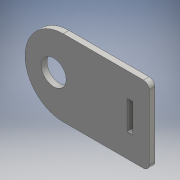
# Autodesk Inventor part: sample_mount
Saved by Autodesk Inventor 2016 (Build 200138000, 138)
## iProperties
Created: 2018-10-08
Part Number: sample_mount
Material: Generic
Document SubType Name: Modeling
Designer: andrew
Density: 1 g/cm^3
Appearance: Default
Author: andrew
Autodesk Inventor part; units mm, degrees
ref_plane "YZ Plane" through (0, 0, 0) normal (1, 0, 0) x (0, 1, 0)
ref_plane "XZ Plane" through (0, 0, 0) normal (0, 1, 0) x (-1, 0, 0)
ref_plane "XY Plane" through (0, 0, 0) normal (0, 0, 1) x (1, 0, 0)
sketch "Sketch1" plane through (0, 0, 0) normal (0, 1, 0) x (-1, 0, 0)
  line L0 (-22.5, 20) -> (22.5, 20)
  line L1 (22.5, 20) -> (22.5, -20)
  line L2 (22.5, -20) -> (-22.5, -20)
  line L3 (-22.5, -20) -> (-22.5, 20)
  line L4 (-22.5, 20) -> (22.5, -20) construction
  line L5 (22.5, 20) -> (-22.5, -20) construction
  arc A0 (22.5, -20) -> (22.5, 20) centre (22.5, 0) ccw
  point P0 (0, 0)
  dimension "d0" = 45
  dimension "d1" = 40
  dimension "d2" = 20
  constraints: 12 end point, 2 midpoint, 2 parallel, 2 point on circle, 1 centre point, 1 horizontal, 1 perpendicular
  measures "d0" distance of L1.end L2.end
  measures "d1" distance of L0.end L1.end
  measures "d2" radius of A0
extrude "Extrusion1" add sketch "Sketch1" along normal blind 3
sketch "Sketch2" plane through (0, 3, 0) normal (0, 1, 0) x (1, 0, 0)
  arc A0 (-22.5, 20) -> (-22.5, -20) centre (-22.5, 0) ccw construction
  line L0 (-42.5, 0) -> (-27.5, 0) construction
  point P0 (0, 0)
  dimension "d5" = 15
  constraints: 2 end point, 1 coincident, 1 horizontal, 1 point on circle
  measures "d5" distance of L0.start L0.end
hole "Hole1" at (-27.5, 3, 0) direction (0, -1, 0) diameter 13 end through all
sketch "Sketch4" plane through (0, 0, 0) normal (0, -1, 0) x (1, 0, 0)
  line L0 (22.5, 20) -> (22.5, -20) construction
  line L1 (22.5, 0) -> (12.5, 0) construction
  line L2 (11, -7.5) -> (14, -7.5)
  line L3 (14, -7.5) -> (14, 7.5)
  line L4 (14, 7.5) -> (11, 7.5)
  line L5 (11, 7.5) -> (11, -7.5)
  line L6 (11, -7.5) -> (14, 7.5) construction
  line L7 (14, -7.5) -> (11, 7.5) construction
  point P0 (0, 0)
  dimension "d17" = 10
  dimension "d18" = 3
  dimension "d19" = 15
  constraints: 14 end point, 3 midpoint, 2 horizontal, 2 parallel, 1 perpendicular
  measures "d17" distance of L1.start L1.end
  measures "d18" distance of L4.end L3.end
  measures "d19" distance of L3.end L2.end
extrude "Extrusion3" cut sketch "Sketch4" against normal blind 10
fillet "Fillet1" radius 3 2 edges at (22.5, 1.5, -20) (22.5, 1.5, 20)
body "Solid1"
